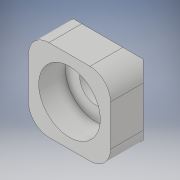
# Autodesk Inventor part: testswitch
Saved by Autodesk Inventor 2017 SP1 (Build 210196100, 196)
## iProperties
Created: 2016-12-24
Part Number: testswitch
Material: Generic
Document SubType Name: Modeling
Designer: wsh32
Density: 1 g/cm^3
Appearance: Default
Author: wsh32
Autodesk Inventor part; units mm, degrees
ref_plane "YZ Plane" through (0, 0, 0) normal (1, 0, 0) x (0, 1, 0)
ref_plane "XZ Plane" through (0, 0, 0) normal (0, 1, 0) x (-1, 0, 0)
ref_plane "XY Plane" through (0, 0, 0) normal (0, 0, 1) x (1, 0, 0)
sketch "Sketch1" plane through (0, 0, 0) normal (0, 0, 1) x (1, 0, 0)
  line L0 (0, 0) -> (12.7, 0)
  line L1 (12.7, 0) -> (12.7, 12.7)
  line L2 (12.7, 12.7) -> (0, 12.7)
  line L3 (0, 12.7) -> (0, 0)
  dimension "d0" = 12.7
  dimension "d1" = 12.7
  constraints: 8 end point, 2 parallel, 1 horizontal, 1 perpendicular
  measures "d0" distance of L2.end L0.start
  measures "d1" distance of L0.start L0.end
extrude "Extrusion1" add sketch "Sketch1" along normal blind 6.35
sketch "Sketch2" plane through (0, 0, 6.35) normal (0, 0, 1) x (1, 0, 0)
  line L0 (0, 12.7) -> (0, 0) construction
  line L1 (0, 0) -> (12.7, 0) construction
  line L2 (0, 12.7) -> (12.7, 0) construction
  line L3 (12.7, 12.7) -> (0, 12.7) construction
  line L4 (0, 0) -> (12.7, 12.7) construction
  point P0 (6.35, 6.35)
  constraints: 4 end point, 1 midpoint
hole "Hole1" at (6.35, 6.35, 6.35) direction (0, 0, -1) diameter 5.08 end through all counterbore diameter 9.525 counterbore depth 4.1275
chamfer "Chamfer1" distance 1.27 angle 45 4 edges at (12.7, 6.35, 0) (6.35, 12.7, 0) (0, 6.35, 0) (6.35, 0, 0)
fillet "Fillet1" radius 3.175 4 edges at (12.7, 12.7, 3.81) (12.7, 0, 3.81) (0, 12.7, 3.81) (0, 0, 3.81)
body "Solid1"
